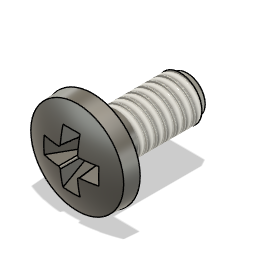
ID_Exam_KhangBui v12 (Autodesk Fusion 360 archive; units mm, degrees)
design "Type II Cross Recessed Binding Head Machine Screw ANSI B18.6.3 0-80 UNF x 0.125 Steel Grade 2 Plain"
description: Type II Cross Recessed Binding Head Machine Screw ANSI B18.6.3 0-80 UNF x 0.125
Autodesk Fusion 360 part; units mm, degrees
sketch "Sketch1" plane through (0, 0, 0) normal (0, 1, 0) x (1, 0, 0)
  line L0 (-0.762, 0) -> (-0.762, 3.175)
  line L1 (-0.762, 3.175) -> (0, 3.175)
  line L2 (0, 3.175) -> (0, -0.8128)
  line L3 (-0.762, 0) -> (-1.6002, 0)
  line L4 (-1.6002, 0) -> (-1.5558, -0.508)
  arc A0 (-1.5558, -0.508) -> (0, -0.8128) centre (0, 3.31) ccw
  dimension "d9" = 1.524
  dimension "d66" = 3.2004
  dimension "d67" = 0.8128
  dimension "d68" = 3.175
  dimension "d143" = 0.3048
  dimension "d146" = 5
  constraint perpendicular L0 L1
  constraint collinear origin L2.end L1.end
  constraint perpendicular L0 L3
  constraint coincident origin L3
  constraint vertical L0
  constraint vertical L2
  constraint coincident L2 A0.centre
  measures "d67" vertical distance of L2.end L3.end
  measures "d68" distance of origin L1.end
  measures "d143" vertical distance of L2.end L4.end
  measures "d146" angle of L2 L4
revolve "Revolve1" add sketch "Sketch1" angle 360 about axis through (0, 0, -3.175) along (0, 0, 1) makes body 1
ref_plane "WorkPlane1" through (0, 0, 0.8128) normal (0, 0, 1) x (1, 0, 0)
sketch "Sketch2" plane through (0, 0, 0.8128) normal (0, 0, 1) x (1, 0, 0)
  line L0 (-0.2921, -0.2921) -> (-0.9906, -0.2921)
  line L1 (-0.2921, -0.9906) -> (-0.2921, -0.2921)
  circle A0 centre (0, 0) radius 0.9906 construction
  line L2 (-0.9906, -0.2921) -> (-0.9906, 0)
  line L3 (-0.9906, 0) -> (0, 0) construction
  line L4 (0, -0.9906) -> (-0.2921, -0.9906)
  line L5 (0, 0) -> (0, -0.9906) construction
  line L6 (0.2921, -0.9906) -> (0, -0.9906)
  line L7 (0.2921, -0.2921) -> (0.2921, -0.9906)
  line L8 (0.9906, -0.2921) -> (0.2921, -0.2921)
  line L9 (0.9906, 0) -> (0.9906, -0.2921)
  line L10 (0.9906, 0.2921) -> (0.9906, 0)
  line L11 (0.2921, 0.2921) -> (0.9906, 0.2921)
  line L12 (0.2921, 0.9906) -> (0.2921, 0.2921)
  line L13 (0, 0.9906) -> (0.2921, 0.9906)
  line L14 (-0.2921, 0.9906) -> (0, 0.9906)
  line L15 (-0.2921, 0.2921) -> (-0.2921, 0.9906)
  line L16 (-0.9906, 0.2921) -> (-0.2921, 0.2921)
  line L17 (-0.9906, 0) -> (-0.9906, 0.2921)
  dimension "d126" = 1.9812
  dimension "d127" = 0.2921
  dimension "d128" = 0.2921
  dimension "d136" = 360
  constraint coincident A0.centre L3.end
  constraint coincident L4.start A0
  constraint vertical L5
  constraint parallel L1 L5
  constraint perpendicular L0 L5
  constraint perpendicular L0 L2
  constraint perpendicular L3 L5
  constraint coincident L2.end A0
  constraint perpendicular L4 L5
  constraint coincident L0.start L1.end
  measures "d126" diameter of A0
  measures "d127" distance of L1.start L4.start
  measures "d128" distance of L0.end L2.end
extrude "Extrude2" add sketch "Sketch2" against normal blind 0.9144 draft -4 separate body makes body 2
draft "Draft2" angle -30 neutral plane through (0, 0, 0.8128) pull (0, 0, 1) 8 faces at (-0.1734, 0.9693, 0.508) (0.1734, 0.9693, 0.508) (0.9693, 0.1734, 0.508) (0.9693, -0.1734, 0.508) (-0.9693, -0.1734, 0.508) (-0.9693, 0.1734, 0.508) (0.1734, -0.9693, 0.508) (-0.1734, -0.9693, 0.508) on bodies 2
fillet "Fillet5" radius 0.0594 4 edges at (-0.2601, -0.2601, 0.3556) (0.2601, -0.2601, 0.3556) (0.2601, 0.2601, 0.3556) (-0.2601, 0.2601, 0.3556) on bodies 2
combine "Combine1" operation cut target body 1 tool bodies 2
thread "Thread2" "ANSI Unified Screw Threads 0.06(#0) 0-80 UNF 2A" major diameter 1.4707 minor diameter 1.1328 pitch 0.3175 angle 60 resizes the face on face at (-0.7611, 0.038, -2.1167) from (0, 0, -0.7937) to (0, 0, -3.175) on bodies 1
sketch "Sketch5" plane through (0, 0, 0) normal (0, 1, 0) x (1, 0, 0)
  line L0 (0, 3.175) -> (0, -0.8128)
  line L1 (0, 3.175) -> (-0.7772, 3.175)
  line L2 (-0.7772, 3.175) -> (-0.7772, 2.8575)
  line L3 (-0.7772, 2.8575) -> (-0.6032, 3.175)
  dimension "d100" = 0.7772
  dimension "d101" = 0.6033
  dimension "d102" = 0.3175
  constraint coincident L0.start L1.start
  constraint perpendicular L0 L1
  constraint perpendicular L1 L2
  constraint coincident L1 L3.end
  measures "d100" horizontal distance of origin L1.end
  measures "d101" horizontal distance of origin L3.end
  measures "d102" distance of L1.end L2.end
revolve "Revolve2" cut sketch "Sketch5" angle 360 about axis through (0, 0, 1.75) along (0, 0, 1) bodies 1
equation "d9 = adsk_nomdia"
equation "d66 = adsk_headdia"
equation "d67 = adsk_headh"
equation "d68 = adsk_nomlen"
equation "d71 = adsk_headh"
equation "adsk_nomlen = 0.125 in"
equation "adsk_headh = 0.032 in"
equation "adsk_headdia = 0.126 in"
equation "adsk_nomdia = 0.06 in"
equation "adsk_phildia = 0.078 in"
equation "adsk_philwidth = 0.023 in"
equation "adsk_phildepth = 0.036 in"
equation "adsk_thrlen = 0.09375 in"
equation "d84 = adsk_thrlen"
equation "adsk_startlen = 0.0125 in"
equation "adsk_endpointdia = 0.0475 in"
equation "d100 = adsk_nomdia * 0.51"
equation "d101 = adsk_endpointdia / 2"
equation "d102 = adsk_startlen"
equation "d126 = adsk_phildia"
equation "d127 = adsk_philwidth / 2"
equation "d128 = adsk_philwidth / 2"
equation "d137 = -adsk_phildepth"
equation "d142 = adsk_phildia * 0.03"
equation "d143 = adsk_ovalh"
equation "adsk_ovalh = 0.012 in"
equation "adsk_headang = 5.00 deg"
equation "d146 = adsk_headang"
